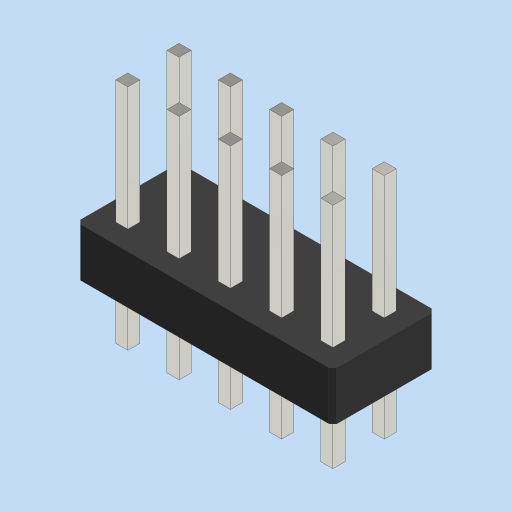
# Autodesk Inventor part: 2x5_P2.54mm_male_header
Saved by Autodesk Inventor 2024 (Build 280153000, 153)
## iProperties
Created: 2025-05-08
Part Number: 2x5_P2.54mm_male_header
Material: Generic
Document SubType Name: Modeling
Designer: XxPan
Density: 1 g/cm^3
Appearance: Default
Author: XxPan
Autodesk Inventor part; units mm, degrees
ref_plane "YZ Plane" through (0, 0, 0) normal (1, 0, 0) x (0, 1, 0)
ref_plane "XZ Plane" through (0, 0, 0) normal (0, 1, 0) x (-1, 0, 0)
ref_plane "XY Plane" through (0, 0, 0) normal (0, 0, 1) x (1, 0, 0)
sketch "Sketch1" plane through (0, 0, 0) normal (0, 1, 0) x (-1, 0, 0)
  line L0 (0, 0) -> (12.7, 0)
  line L1 (12.7, 0) -> (12.7, -5.08)
  line L2 (12.7, -5.08) -> (0, -5.08)
  line L3 (0, -5.08) -> (0, 0)
  dimension "d0" = 12.7
  dimension "d1" = 5.08
  constraints: 8 end point, 2 parallel, 1 horizontal, 1 perpendicular
  measures "d0" distance of L1.end L2.end
  measures "d1" distance of L0.end L1.end
extrude "Extrusion1" add sketch "Sketch1" along normal blind 2.4
chamfer "Chamfer1" distance 0.2 angle 45 4 edges at (-12.7, 1.2, -5.08) (-12.7, 1.2, 0) (0, 1.2, 0) (0, 1.2, -5.08)
sketch "Sketch2" plane through (0, 2.4, 0) normal (0, 1, 0) x (1, 0, 0)
  line L0 (-11.13, 0.97) -> (-11.73, 0.97)
  line L1 (-11.73, 0.97) -> (-11.73, 1.57)
  line L2 (-11.73, 1.57) -> (-11.13, 1.57)
  line L3 (-11.13, 1.57) -> (-11.13, 0.97)
  line L4 (-11.13, 0.97) -> (-11.73, 1.57) construction
  line L5 (-11.73, 0.97) -> (-11.13, 1.57) construction
  line L6 (-11.13, 3.51) -> (-11.73, 3.51)
  line L7 (-11.73, 3.51) -> (-11.73, 4.11)
  line L8 (-11.73, 4.11) -> (-11.13, 4.11)
  line L9 (-11.13, 4.11) -> (-11.13, 3.51)
  line L10 (-11.13, 3.51) -> (-11.73, 4.11) construction
  line L11 (-11.73, 3.51) -> (-11.13, 4.11) construction
  line L12 (-8.59, 0.97) -> (-9.19, 0.97)
  line L13 (-9.19, 0.97) -> (-9.19, 1.57)
  line L14 (-9.19, 1.57) -> (-8.59, 1.57)
  line L15 (-8.59, 1.57) -> (-8.59, 0.97)
  line L16 (-8.59, 0.97) -> (-9.19, 1.57) construction
  line L17 (-9.19, 0.97) -> (-8.59, 1.57) construction
  line L18 (-8.59, 3.51) -> (-9.19, 3.51)
  line L19 (-9.19, 3.51) -> (-9.19, 4.11)
  line L20 (-9.19, 4.11) -> (-8.59, 4.11)
  line L21 (-8.59, 4.11) -> (-8.59, 3.51)
  line L22 (-8.59, 3.51) -> (-9.19, 4.11) construction
  line L23 (-9.19, 3.51) -> (-8.59, 4.11) construction
  line L24 (-6.05, 0.97) -> (-6.65, 0.97)
  line L25 (-6.65, 0.97) -> (-6.65, 1.57)
  line L26 (-6.65, 1.57) -> (-6.05, 1.57)
  line L27 (-6.05, 1.57) -> (-6.05, 0.97)
  line L28 (-6.05, 0.97) -> (-6.65, 1.57) construction
  line L29 (-6.65, 0.97) -> (-6.05, 1.57) construction
  line L30 (-6.05, 3.51) -> (-6.65, 3.51)
  line L31 (-6.65, 3.51) -> (-6.65, 4.11)
  line L32 (-6.65, 4.11) -> (-6.05, 4.11)
  line L33 (-6.05, 4.11) -> (-6.05, 3.51)
  line L34 (-6.05, 3.51) -> (-6.65, 4.11) construction
  line L35 (-6.65, 3.51) -> (-6.05, 4.11) construction
  line L36 (-3.51, 0.97) -> (-4.11, 0.97)
  line L37 (-4.11, 0.97) -> (-4.11, 1.57)
  line L38 (-4.11, 1.57) -> (-3.51, 1.57)
  line L39 (-3.51, 1.57) -> (-3.51, 0.97)
  line L40 (-3.51, 0.97) -> (-4.11, 1.57) construction
  line L41 (-4.11, 0.97) -> (-3.51, 1.57) construction
  line L42 (-3.51, 3.51) -> (-4.11, 3.51)
  line L43 (-4.11, 3.51) -> (-4.11, 4.11)
  line L44 (-4.11, 4.11) -> (-3.51, 4.11)
  line L45 (-3.51, 4.11) -> (-3.51, 3.51)
  line L46 (-3.51, 3.51) -> (-4.11, 4.11) construction
  line L47 (-4.11, 3.51) -> (-3.51, 4.11) construction
  line L48 (-0.97, 0.97) -> (-1.57, 0.97)
  line L49 (-1.57, 0.97) -> (-1.57, 1.57)
  line L50 (-1.57, 1.57) -> (-0.97, 1.57)
  line L51 (-0.97, 1.57) -> (-0.97, 0.97)
  line L52 (-0.97, 0.97) -> (-1.57, 1.57) construction
  line L53 (-1.57, 0.97) -> (-0.97, 1.57) construction
  line L54 (-0.97, 3.51) -> (-1.57, 3.51)
  line L55 (-1.57, 3.51) -> (-1.57, 4.11)
  line L56 (-1.57, 4.11) -> (-0.97, 4.11)
  line L57 (-0.97, 4.11) -> (-0.97, 3.51)
  line L58 (-0.97, 3.51) -> (-1.57, 4.11) construction
  line L59 (-1.57, 3.51) -> (-0.97, 4.11) construction
  line L60 (-12.7, 4.88) -> (-12.7, 0.2) projected
  line L61 (-12.5, 0) -> (-0.2, 0) projected
  point P0 (0, 0)
  point P1 (-11.43, 1.27)
  point P2 (-11.43, 3.81)
  point P3 (-8.89, 1.27)
  point P4 (-8.89, 3.81)
  point P5 (-6.35, 1.27)
  point P6 (-6.35, 3.81)
  point P7 (-3.81, 1.27)
  point P8 (-3.81, 3.81)
  point P9 (-1.27, 1.27)
  point P10 (-1.27, 3.81)
  dimension "d7" = 0.6
  dimension "d8" = 0.6
  dimension "d11" = 2.54
  dimension "d14" = 2.54
  dimension "d17" = 1.27
  dimension "d18" = 1.27
  constraints: 120 end point, 2 collinear, 2 horizontal, 2 midpoint, 2 parallel, 1 perpendicular, 1 vertical, 97 other
  measures "d7" distance of L1.end L2.end
  measures "d8" distance of L0.end L1.end
  measures "d11" distance of L0.start L6.start
  measures "d14" distance of L0.start L12.start
  measures "d17" distance from line of L60 point (-11.43, 1.27)
  measures "d18" distance from line of L61 point (-11.43, 1.27)
extrude "Extrusion2" add sketch "Sketch2" along normal blind 6.1 and the other way blind 5.2
body "Solid1"
